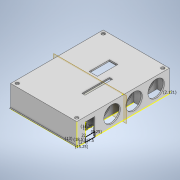
# Autodesk Inventor part: upper casing
Saved by Autodesk Inventor 2020 (Build 240168000, 168)
## iProperties
Created: 2019-06-23
Part Number: upper casing
Material: Generic
Document SubType Name: Modeling
Designer: jjsch
Density: 1 g/cm^3
Appearance: Default
Mass: 107.508 g
Surface Area: 832.789 cm^2
Volume: 107.508 cm^3
Author: jjsch
Autodesk Inventor part; units mm, degrees
ref_plane "YZ Plane" through (0, 0, 0) normal (1, 0, 0) x (0, 1, 0)
ref_plane "XZ Plane" through (0, 0, 0) normal (0, 1, 0) x (-1, 0, 0)
ref_plane "XY Plane" through (0, 0, 0) normal (0, 0, 1) x (1, 0, 0)
sketch "Sketch1" plane through (0, 0, 0) normal (0, 1, 0) x (-1, 0, 0)
  line L0 (-1.2, -80) -> (1.2, -80)
  line L1 (1.2, -80) -> (1.2, 80)
  line L2 (1.2, 80) -> (-1.2, 80)
  line L3 (-1.2, 80) -> (-1.2, -80)
  line L4 (-1.2, -80) -> (1.2, 80) construction
  line L5 (1.2, -80) -> (-1.2, 80) construction
  point P0 (0, 0)
  dimension "d0" = 2.4
  dimension "d1" = 160
  constraints: 12 end point, 2 midpoint, 2 parallel, 1 horizontal, 1 perpendicular
  measures "d0" distance of L2.end L1.end
  measures "d1" distance of L1.end L0.end
extrude "Extrusion1" add sketch "Sketch1" along normal blind 40
sketch "Sketch2" plane through (1.2, 0, 80) normal (1, 0, 0) x (0, 0, -1)
  line L0 (0, 0) -> (0, 40) projected
  line L1 (160, 0) -> (160, 40) projected
  circle A0 centre (60, 20) radius 15
  circle A1 centre (100, 20) radius 15
  circle A2 centre (140, 20) radius 15
  line L2 (28.75, 31.75) -> (11.25, 31.75)
  line L3 (11.25, 31.75) -> (11.25, 8.25)
  line L4 (11.25, 8.25) -> (28.75, 8.25)
  line L5 (28.75, 8.25) -> (28.75, 31.75)
  line L6 (28.75, 31.75) -> (11.25, 8.25) construction
  line L7 (11.25, 31.75) -> (28.75, 8.25) construction
  point P0 (80, 0)
  point P1 (20, 20)
  dimension "d4" = 60
  dimension "d5" = 20
  dimension "d6" = 40
  dimension "d7" = 20
  dimension "d8" = 30
  dimension "d9" = 30
  dimension "d10" = 30
  dimension "d11" = 17.5
  dimension "d12" = 23.5
  constraints: 12 end point, 3 centre point, 3 coincident, 2 midpoint, 2 parallel, 1 horizontal, 1 perpendicular
  measures "d4" distance from line of L0 point (60, 20)
  measures "d5" distance from line of L1 point (140, 20)
  measures "d6" distance of point (140, 20) point (100, 20)
  measures "d7" distance from line of L0 point (20, 20)
  measures "d8" diameter of A0
  measures "d9" diameter of A1
  measures "d10" diameter of A2
  measures "d11" distance of L4.end L3.end
  measures "d12" distance of L3.end L2.end
extrude "Extrusion2" cut sketch "Sketch2" against normal blind 40
sketch "Sketch3" plane through (1.2, 0, -80) normal (0, 0, -1) x (-1, 0, 0)
  line L0 (2.4, 0) -> (2.4, 40) projected
  point P0 (1.2, 0)
sketch "Sketch4" plane through (0, 40, 0) normal (0, 1, 0) x (1, 0, 0)
  line L0 (1.2, -80) -> (-118.8, -80)
  line L1 (-118.8, -80) -> (-118.8, 80)
  line L2 (-118.8, 80) -> (1.2, 80)
  line L3 (1.2, 80) -> (1.2, -80)
  point P0 (0, 0)
  dimension "d17" = 120
  dimension "d18" = 160
  constraints: 8 end point, 2 parallel, 1 horizontal, 1 perpendicular
  measures "d17" distance of L1.end L2.end
  measures "d18" distance of L0.end L1.end
extrude "Extrusion3" add sketch "Sketch4" against normal blind 2.4
sketch "Sketch5" plane through (-1.2, 0, -80) normal (-1, 0, 0) x (0, 0, 1)
  circle A0 centre (20, 20) radius 15 projected
  circle A1 centre (60, 20) radius 15 projected
  circle A2 centre (100, 20) radius 15 projected
  line L0 (160, 37.6) -> (0, 37.6) projected
  line L1 (9, 37.6) -> (31, 37.6)
  line L2 (31, 30.198) -> (31, 37.6)
  line L3 (9, 37.6) -> (9, 30.198)
  arc A3 (31, 30.198) -> (9, 30.198) centre (20, 20) ccw
  arc A4 (71, 30.198) -> (49, 30.198) centre (60, 20) ccw
  arc A5 (111, 30.198) -> (89, 30.198) centre (100, 20) ccw
  line L4 (49, 30.198) -> (49, 37.6)
  line L5 (49, 37.6) -> (71, 37.6)
  line L6 (71, 37.6) -> (71, 30.198)
  line L7 (89, 30.198) -> (89, 37.6)
  line L8 (89, 37.6) -> (111, 37.6)
  line L9 (111, 37.6) -> (111, 30.198)
  point P0 (80, 0)
  constraints: 18 end point, 12 point on circle, 6 point on line, 5 perpendicular, 3 centre point, 3 concentric, 1 parallel
extrude "Extrusion4" add sketch "Sketch5" along normal blind 28.6 contours A0 L3 L0 L2 | A1 L4 L0 L6 | A2 L7 L0 L9
sketch "Sketch6" plane through (-1.2, 0, -80) normal (-1, 0, 0) x (0, 0, 1)
  point P0 (80, 0)
sketch "Sketch7" plane through (-1.2, 0, -80) normal (-1, 0, 0) x (0, 0, 1)
  line L0 (160, 0) -> (160, 37.6) projected
  line L1 (129.75, 33.25) -> (129.75, 8.25)
  line L2 (129.75, 8.25) -> (150.25, 8.25)
  line L3 (150.25, 8.25) -> (150.25, 33.25)
  line L4 (151.5882, 33.25) -> (128.5882, 33.25)
  line L5 (131.25, 31.75) -> (148.75, 31.75) projected
  line L6 (150.25, 33.25) -> (129.75, 33.25)
  line L7 (151.25, 34.25) -> (151.25, 7.25)
  line L8 (151.25, 7.25) -> (128.75, 7.25)
  line L9 (128.75, 7.25) -> (128.75, 34.25)
  line L10 (128.75, 34.25) -> (151.25, 34.25)
  line L11 (148.75, 8.25) -> (131.25, 8.25) projected
  line L12 (131.25, 8.25) -> (131.25, 31.75) projected
  line L13 (148.75, 31.75) -> (148.75, 8.25) projected
  point P0 (80, 0)
  point P1 (129.75, 33.25)
  dimension "d25" = 20.5
  dimension "d26" = 25
  dimension "d27" = 23
  dimension "d129" = 1
  dimension "d158" = 1.5
  dimension "d159" = 1.5
  dimension "d160" = 1.5
  constraints: 18 end point, 2 parallel, 1 horizontal, 3 other
  measures "d25" distance of L2.end L1.end
  measures "d26" distance of L1.end L1.start
  measures "d27" distance of L4.end L4.start
  measures "d129" distance between parallel lines of L3 L7
  measures "d158" distance between parallel lines of L5 L6
  measures "d159" distance between parallel lines of L12 L1
  measures "d160" distance between parallel lines of L3 L13
extrude "Extrusion5" add sketch "Sketch7" along normal blind 1.5 contours L4 L9 L10 L7 | L1 L2 L3 L4 L7 L8 L9
sketch "Sketch12" plane through (1.2, 0, -80) normal (0, 0, -1) x (-1, 0, 0)
  line L0 (0, 40) -> (120, 40) projected
  line L1 (0, 40) -> (120, 40)
  line L2 (120, 40) -> (120, 0)
  line L3 (120, 0) -> (0, 0)
  line L4 (0, 0) -> (0, 40)
  point P0 (1.2, 0)
  dimension "d96" = 120
  constraints: 8 end point, 2 parallel, 1 horizontal, 1 perpendicular
  measures "d96" distance of L2.end L3.end
extrude "Extrusion10" add sketch "Sketch12" along normal blind 4
sketch "Sketch13" plane through (0, 37.6, 0) normal (0, -1, 0) x (1, 0, 0)
  point P0 (0, 0)
sketch "Sketch14" plane through (1.2, 0, 80) normal (0, 0, 1) x (1, 0, 0)
  line L0 (-120, 40) -> (-120, 37.6) projected
  line L1 (-2.4, 0) -> (0, 0) projected
  line L2 (-120, 40) -> (0, 40)
  line L3 (0, 40) -> (0, 0)
  line L4 (0, 0) -> (-120, 0)
  line L5 (-120, 0) -> (-120, 40)
  point P0 (-1.2, 0)
  constraints: 8 end point, 2 parallel, 1 horizontal, 1 perpendicular
extrude "Extrusion11" add sketch "Sketch14" along normal blind 4
sketch "Sketch15" plane through (1.2, 0, 68.75) normal (1, 0, 0) x (0, 0, -1)
  point P0 (68.75, 0)
sketch "Sketch16" plane through (0, 37.6, 0) normal (0, -1, 0) x (1, 0, 0)
  line L0 (-1.2, 80) -> (-118.8, 80) projected
  line L1 (-22.3, 80) -> (-17.3, 80)
  line L2 (-17.3, 80) -> (-17.3, -80)
  line L3 (-17.3, -80) -> (-22.3, -80)
  line L4 (-22.3, -80) -> (-22.3, 80)
  point P0 (0, 0)
  dimension "d47" = 5
  dimension "d48" = 160
  constraints: 8 end point, 2 parallel, 1 horizontal, 1 perpendicular, 1 point on line
  measures "d47" distance of L2.end L3.end
  measures "d48" distance of L1.end L2.end
extrude "Extrusion12" add sketch "Sketch16" along normal up to surface (37.6 mm away)
sketch "Sketch18" plane through (1.2, 0, 68.75) normal (1, 0, 0) x (0, 0, -1)
  point P0 (68.75, 0)
sketch "Sketch21" plane through (0, 37.6, 0) normal (0, -1, 0) x (1, 0, 0)
  line L0 (-1.2, -80) -> (-1.2, 80) projected
  line L1 (-17.3, -80) -> (-17.3, 80) projected
  line L2 (-1.2, -49) -> (-17.3, -49) projected
  line L3 (-1.2, -31) -> (-17.3, -31) projected
  line L4 (-17.3, -38) -> (-1.2, -38)
  line L5 (-1.2, -38) -> (-1.2, -42)
  line L6 (-1.2, -42) -> (-17.3, -42)
  line L7 (-17.3, -42) -> (-17.3, -38)
  line L8 (-17.3, -38) -> (-1.2, -42) construction
  line L9 (-1.2, -38) -> (-17.3, -42) construction
  point P0 (0, 0)
  point P1 (-9.25, -40)
  point P2 (-1.2, -2)
  point P3 (-17.3, -2)
  point P4 (-1.2, -38)
  dimension "d59" = 8.05
  dimension "d60" = 8.05
  dimension "d61" = 9
  dimension "d62" = 9
  dimension "d63" = 16.1
  dimension "d64" = 4
  constraints: 12 end point, 2 midpoint, 2 parallel, 1 horizontal, 1 perpendicular
  measures "d59" distance from line of L0 point (-9.25, -40)
  measures "d60" distance from line of L1 point (-9.25, -40)
  measures "d61" distance from line of L2 point (-9.25, -40)
  measures "d62" distance from line of L3 point (-9.25, -40)
  measures "d63" distance of L5.end L6.end
  measures "d64" distance of L4.end L5.end
extrude "Extrusion16" add sketch "Sketch21" along normal up to surface (37.6 mm away) contours L6 L1 L4 L0
sketch "Sketch22" plane through (0, 37.6, 0) normal (0, -1, 0) x (1, 0, 0)
  point P0 (0, 0)
sketch "Sketch23" plane through (0, 37.6, 0) normal (0, -1, 0) x (1, 0, 0)
  line L0 (-118.8, 80) -> (-118.8, -80) projected
  line L1 (-22.3, 80) -> (-118.8, 80) projected
  circle A0 centre (-66.3, 76.5) radius 3
  circle A1 centre (-115.3, 76.5) radius 3
  circle A2 centre (-115.3, 18.5) radius 3
  circle A3 centre (-66.3, 18.5) radius 3
  circle A4 centre (-66.3, 18.5) radius 1.375
  circle A5 centre (-115.3, 18.5) radius 1.375
  circle A6 centre (-115.3, 76.5) radius 1.375
  circle A7 centre (-66.3, 76.5) radius 1.375
  point P0 (0, 0)
  dimension "d67" = 58
  dimension "d68" = 58
  dimension "d69" = 49
  dimension "d70" = 3.5
  dimension "d71" = 3.5
  dimension "d72" = 6
  dimension "d73" = 6
  dimension "d74" = 6
  dimension "d75" = 6
  dimension "d78" = 2.75
  dimension "d79" = 2.75
  dimension "d80" = 2.75
  dimension "d81" = 2.75
  constraints: 8 centre point, 8 coincident, 2 vertical alignment, 1 horizontal alignment
  measures "d67" distance of point (-66.3, 18.5) point (-66.3, 76.5)
  measures "d68" distance of point (-115.3, 18.5) point (-115.3, 76.5)
  measures "d69" distance of point (-66.3, 18.5) point (-115.3, 18.5)
  measures "d70" distance from line of L0 point (-115.3, 76.5)
  measures "d71" distance from line of L1 point (-115.3, 76.5)
  measures "d72" diameter of A0
  measures "d73" diameter of A1
  measures "d74" diameter of A2
  measures "d75" diameter of A3
  measures "d78" diameter of A4
  measures "d79" diameter of A5
  measures "d80" diameter of A6
  measures "d81" diameter of A7
extrude "Extrusion17" add sketch "Sketch23" along normal blind 8
sketch "Sketch28" plane through (0, 0, 0) normal (0, -1, 0) x (1, 0, 0)
  point P0 (0, 0)
sketch "Sketch29" plane through (0, 37.6, 0) normal (0, -1, 0) x (1, 0, 0)
  circle A0 centre (-115.3, 18.5) radius 3 projected
  circle A1 centre (-66.3, 18.5) radius 3 projected
  circle A2 centre (-115.3, 76.5) radius 3 projected
  circle A3 centre (-66.3, 76.5) radius 3 projected
  line L0 (-1.2, -71) -> (-17.3, -71) projected
  line L1 (-29.8, -71) -> (-29.8, -49) projected
  line L2 (-29.8, -49) -> (-22.3, -49) projected
  line L3 (-1.2, -31) -> (-17.3, -31) projected
  line L4 (-29.8, -31) -> (-29.8, -9) projected
  line L5 (-29.8, -9) -> (-22.3, -9) projected
  line L6 (-1.2, 9) -> (-17.3, 9) projected
  line L7 (-29.8, 9) -> (-29.8, 31) projected
  line L8 (-29.8, 31) -> (-22.3, 31) projected
  line L9 (-1.2, 80) -> (-17.3, 80) projected
  line L10 (-118.8, 80) -> (-118.8, -80) projected
  line L11 (-118.8, -80) -> (-22.3, -80) projected
  line L12 (-35.8, -3) -> (-35.8, -37)
  line L13 (-35.8, -37) -> (-28.3, -37)
  line L14 (-28.3, -37) -> (-28.3, -43)
  line L15 (-28.3, -43) -> (-35.8, -43)
  line L16 (-35.8, -43) -> (-35.8, -74)
  line L17 (-35.8, -74) -> (-112.8, -74)
  line L18 (-112.8, -74) -> (-112.8, 74)
  line L19 (-112.8, 74) -> (-28.3, 74)
  line L20 (-28.3, 74) -> (-28.3, 37)
  line L21 (-28.3, 37) -> (-35.8, 37)
  line L22 (-35.8, 37) -> (-35.8, 3)
  line L23 (-35.8, 3) -> (-28.3, 3)
  line L24 (-28.3, 3) -> (-28.3, -3)
  line L25 (-28.3, -3) -> (-35.8, -3)
  line L26 (-112.8, -74) -> (-35.8, -74)
  line L27 (-35.8, -74) -> (-35.8, -6)
  line L28 (-35.8, -6) -> (-112.8, -6)
  line L29 (-112.8, -6) -> (-112.8, -74)
  line L30 (-66.3, -74) -> (-51.3, -74)
  line L31 (-51.3, -74) -> (-51.3, -6)
  line L32 (-51.3, -6) -> (-66.3, -6)
  line L33 (-66.3, -6) -> (-66.3, -74)
  line L34 (-51.3, -51.2056) -> (-36.3, -51.2056) construction
  line L35 (-118.8, -84) -> (1.2, -84) projected
  line L36 (-59.1553, -43) -> (-66.3, -43)
  line L37 (-59.1553, -43) -> (-51.3, -43)
  line L38 (-142.8, 0) -> (25.2, 0) projected
  line L39 (-17.3, 31) -> (-1.2, 31) projected
  line L40 (-1.2, -42) -> (-17.3, -42) projected
  line L41 (-17.3, -42) -> (-17.3, -49) projected
  line L42 (-17.3, -49) -> (-1.2, -49) projected
  line L43 (-1.2, -42) -> (-1.2, -49) projected
  line L44 (-17.3, -71) -> (-17.3, -80) projected
  line L45 (-17.3, -80) -> (-1.2, -80) projected
  line L46 (-1.2, -71) -> (-1.2, -80) projected
  line L47 (-17.3, 80) -> (-17.3, 31) projected
  line L48 (-17.3, -9) -> (-1.2, -9) projected
  line L49 (-1.2, 9) -> (-1.2, -9) projected
  line L50 (-1.2, 80) -> (-1.2, 31) projected
  line L51 (-17.3, 9) -> (-17.3, -9) projected
  line L52 (-17.3, -38) -> (-1.2, -38) projected
  line L53 (-1.2, -31) -> (-1.2, -38) projected
  line L54 (-17.3, -31) -> (-17.3, -38) projected
  line L55 (-22.3, 80) -> (-118.8, 80) projected
  line L56 (-22.3, -71) -> (-29.8, -71) projected
  line L57 (-22.3, -31) -> (-29.8, -31) projected
  line L58 (-22.3, 9) -> (-29.8, 9) projected
  line L59 (-22.3, 31) -> (-22.3, 80) projected
  line L60 (-22.3, -80) -> (-22.3, -71) projected
  line L61 (-22.3, -49) -> (-22.3, -31) projected
  line L62 (-22.3, -9) -> (-22.3, 9) projected
  point P0 (0, 0)
  point P1 (-66.3, -6)
  dimension "d97" = 6
  dimension "d98" = 15
  dimension "d110" = 41
  dimension "d118" = 6
  constraints: 50 end point, 6 point on line, 4 parallel, 3 horizontal, 3 perpendicular, 7 other
  measures "d97" distance between parallel lines of L4 L12
  measures "d98" distance of L32.end L31.end
  measures "d110" distance from line of L35 L36.start
  measures "d118" distance between parallel lines of L38 L28
extrude "Extrusion20" cut sketch "Sketch29" along normal mid plane 10 contours L28 L31 L37 L36 L33
sketch "Sketch30" plane through (0, 40, 0) normal (0, 1, 0) x (1, 0, 0)
  line L0 (-51.3, 43) -> (-51.3, 6) projected
  line L1 (-51.3, 6) -> (-66.3, 6) projected
  line L2 (-66.3, 6) -> (-66.3, 43) projected
  line L3 (1.2, 84) -> (1.2, -84) projected
  line L4 (-118.8, 84) -> (1.2, 84) projected
  line L5 (-118.8, 84) -> (-118.8, -84) projected
  line L6 (1.2, -84) -> (-118.8, -84) projected
  line L7 (-112.8, -78) -> (-112.8, 78)
  line L8 (-112.8, 78) -> (-4.8, 78)
  line L9 (-4.8, 78) -> (-4.8, -78)
  line L10 (-4.8, -78) -> (-112.8, -78)
  circle A0 centre (-112.8, -78) radius 3
  circle A1 centre (-112.8, 78) radius 3
  circle A2 centre (-4.8, -78) radius 3
  circle A3 centre (-4.8, 78) radius 3
  line L11 (-66.3, 43) -> (-51.3, 43) projected
  point P0 (0, 0)
  dimension "d101" = 6
  dimension "d102" = 6
  dimension "d103" = 6
  dimension "d104" = 6
  dimension "d105" = 6
  constraints: 8 coincident, 8 end point, 4 centre point, 3 other
  measures "d101" distance between parallel lines of L6 L10
  measures "d102" diameter of A0
  measures "d103" diameter of A1
  measures "d104" diameter of A2
  measures "d105" diameter of A3
sketch "Sketch31" plane through (0, 40, 0) normal (0, 1, 0) x (1, 0, 0)
  point P0 (0, 0)
extrude "Extrusion21" cut sketch "Sketch30" against normal blind 2 contours L10 A0 L7 | L7 A0 L10 | A1 L8 L7 | L7 L8 A1 | A2 L9 L10 | L10 L9 A2 | A3 L9 L8 | L8 L9 A3
sketch "Sketch32" plane through (0, 40, 0) normal (0, 1, 0) x (1, 0, 0)
  line L0 (1.2, 84) -> (1.2, -84) projected
  line L1 (-118.8, 84) -> (1.2, 84) projected
  line L2 (-32.842, -35) -> (-32.842, 15)
  line L3 (-32.842, 15) -> (-38.382, 15)
  line L4 (-38.382, 15) -> (-38.382, -35)
  line L5 (-38.382, -35) -> (-32.842, -35)
  point P0 (0, 0)
  dimension "d111" = 50
  dimension "d112" = 34.042
  dimension "d113" = 34.042
  dimension "d114" = 69
  dimension "d115" = 5.54
  constraints: 8 end point, 3 perpendicular
  measures "d111" distance of L2.end L2.start
  measures "d112" distance from line of L0 L2.start
  measures "d113" distance from line of L0 L2.end
  measures "d114" distance from line of L1 L2.end
  measures "d115" distance of L2.end L3.end
extrude "Extrusion22" cut sketch "Sketch32" against normal blind 10
sketch "Sketch33" plane through (0, 37.6, 0) normal (0, -1, 0) x (1, 0, 0)
  point P0 (0, 0)
sketch "Sketch34" plane through (0, 40, 0) normal (0, 1, 0) x (1, 0, 0)
  point P0 (0, 0)
sketch "Sketch42" plane through (-17.3, 37.6, 80) normal (1, 0, 0) x (0, 0, -1)
  line L0 (31, -26.35) -> (31, -3.6)
  line L1 (9, -3.6) -> (9, -26.35)
  line L2 (31, -3.6) -> (31, -4.35)
  line L3 (9, -3.6) -> (9, -4.35)
  line L4 (9, -4.35) -> (31, -4.35)
  line L5 (9, -26.35) -> (31, -26.35)
  line L6 (0, 0) -> (49, 0) projected
  line L7 (0, -37.6) -> (0, 0) projected
  line L8 (30.25, -4.35) -> (9.75, -4.35) projected
  line L9 (8.75, -3.35) -> (31.25, -3.35) projected
  point P0 (80, -37.6)
  point P1 (9, -4.35)
  dimension "d162" = 22
  dimension "d163" = 4.35
  dimension "d164" = 9
  dimension "d165" = 22
  dimension "d177" = 1
  constraints: 12 end point, 1 perpendicular, 1 point on line, 1 other
  measures "d162" distance between parallel lines of L5 L4
  measures "d163" distance between parallel lines of L4 L6
  measures "d164" distance between parallel lines of L1 L7
  measures "d165" distance between parallel lines of L0 L1
extrude "Extrusion30" cut sketch "Sketch42" against normal blind 10
sketch "Sketch43" plane through (-17.3, 37.6, 80) normal (1, 0, 0) x (0, 0, -1)
  line L0 (-0.75, -32.95) -> (2.65, -32.95)
  line L1 (2.65, -32.95) -> (2.65, -6.35)
  line L2 (2.65, -6.35) -> (-0.75, -6.35)
  line L3 (-0.75, -6.35) -> (-0.75, -32.95)
  line L4 (4.65, -34.95) -> (-2.75, -34.95)
  line L5 (-2.75, -34.95) -> (-2.75, -4.35)
  line L6 (-2.75, -4.35) -> (4.65, -4.35)
  line L7 (4.65, -4.35) -> (4.65, -34.95)
  line L8 (9, -4.35) -> (31, -4.35) projected
  point P0 (80, -37.6)
  point P1 (0.95, -27.95)
  point P2 (9, -26.35)
  point P3 (-4, -37.6)
  dimension "d168" = 8.05
  dimension "d169" = 1.6
  dimension "d170" = 3.4
  dimension "d172" = 2
  dimension "d173" = 3.25
  dimension "d174" = 1.25
  dimension "d178" = 0
  constraints: 16 end point, 4 parallel, 2 perpendicular, 1 horizontal, 3 other
  measures "d168" horizontal distance of point (0.95, -27.95) point (9, -26.35)
  measures "d169" vertical distance of point (9, -26.35) point (0.95, -27.95)
  measures "d170" distance of L2.end L1.end
  measures "d172" distance between parallel lines of L0 L4
  measures "d173" distance from line of point (-4, -37.6) L3
  measures "d174" distance from line of point (-4, -37.6) L5
  measures "d178" distance between parallel lines of L8 L6
extrude "Extrusion31" cut sketch "Sketch43" along normal mid plane 30 contours L3 L2 L1 L0 | L4 L5 L6 L7
sketch "Sketch44" plane through (-17.3, 37.6, 80) normal (1, 0, 0) x (0, 0, -1)
  circle A0 centre (60, -17.6) radius 15 projected
  circle A1 centre (100, -17.6) radius 15 projected
  circle A2 centre (140, -17.6) radius 15 projected
  point P0 (80, -37.6)
extrude "Extrusion32" cut sketch "Sketch44" against normal blind 30
sketch "Sketch45" plane through (1.2, 0, -84) normal (1, 0, 0) x (0, 0, -1)
  line L0 (-152.75, 31.75) -> (-152.75, 8.25) projected
  line L1 (-46, 0) -> (-164, 0) projected
  line L2 (-152.75, 8.25) -> (-135.25, 8.25)
  line L3 (-135.25, 8.25) -> (-135.25, 0)
  line L4 (-135.25, 0) -> (-152.75, 0)
  line L5 (-152.75, 0) -> (-152.75, 8.25)
  line L6 (-168, 0) -> (-168, 40) projected
  point P0 (-84, 0)
  dimension "d181" = 17.5
  dimension "d184" = 8.25
  dimension "d185" = 15.25
  constraints: 8 end point, 2 parallel, 1 horizontal, 1 perpendicular, 1 point on line
  measures "d181" distance of L3.end L4.end
  measures "d184" distance of L2.end L3.end
  measures "d185" distance from line of L4.end L6
extrude "Extrusion33" cut sketch "Sketch45" against normal blind 30
sketch "Sketch46" plane through (0, 0, 0) normal (0, -1, 0) x (1, 0, 0)
  line L0 (-1.2, 68.75) -> (-1.2, 80) projected
  line L1 (1.2, 84) -> (1.2, 68.75) projected
  point P0 (0, 0)
  dimension "d186" = 2.4
  measures "d186" distance between parallel lines of L0 L1
sketch "Sketch47" plane through (0, 0, 0) normal (0, -1, 0) x (1, 0, 0)
  line L0 (-0.6375, 52.5) -> (0.6375, 52.5)
  line L1 (0.6375, 52.5) -> (0.6375, 50)
  line L2 (0.6375, 50) -> (-0.6375, 50)
  line L3 (-0.6375, 50) -> (-0.6375, 52.5)
  line L4 (1.2, 51.25) -> (-1.2, 51.25) projected
  line L5 (-0.6375, 52.5) -> (0.6375, 50) construction
  line L6 (0.6375, 52.5) -> (-0.6375, 50) construction
  line L7 (-0.6375, 70) -> (0.6375, 70)
  line L8 (0.6375, 70) -> (0.6375, 67.5)
  line L9 (0.6375, 67.5) -> (-0.6375, 67.5)
  line L10 (-0.6375, 67.5) -> (-0.6375, 70)
  line L11 (-1.2, 68.75) -> (1.2, 68.75) projected
  line L12 (-0.6375, 70) -> (0.6375, 67.5) construction
  line L13 (0.6375, 70) -> (-0.6375, 67.5) construction
  point P0 (0, 0)
  point P1 (0, 51.25)
  point P2 (0, 68.75)
  point P3 (0.6375, 51.25)
  point P4 (-0.6375, 51.25)
  point P5 (-0.6375, 68.75)
  point P6 (0.6375, 68.75)
  dimension "d187" = 1.275
  dimension "d188" = 2.5
  dimension "d189" = 1.275
  dimension "d190" = 2.5
  constraints: 24 end point, 6 midpoint, 4 parallel, 2 horizontal, 2 perpendicular
  measures "d187" distance of L1.end L2.end
  measures "d188" distance of L0.end L1.end
  measures "d189" distance of L8.end L9.end
  measures "d190" distance of L7.end L8.end
extrude "Extrusion34" cut sketch "Sketch47" against normal blind 8.25 contours L4 L1 L2 L3 | L7 L8 L11 L10
sketch "Sketch48" plane through (-17.3, 37.6, 80) normal (1, 0, 0) x (0, 0, -1)
  line L0 (31, -4.35) -> (31, -26.35) projected
  line L1 (9, -26.35) -> (9, -4.35) projected
  line L2 (9, -4.35) -> (9, -26.35) projected
  line L3 (118, -37.6) -> (28.75, -37.6) projected
  line L4 (9, -26.35) -> (31, -26.35)
  line L5 (31, -26.35) -> (31, -37.6)
  line L6 (31, -37.6) -> (9, -37.6)
  line L7 (9, -37.6) -> (9, -26.35)
  point P0 (80, -37.6)
  point P1 (28.75, -37.6)
  dimension "d193" = 11.25
  dimension "d194" = 22
  constraints: 8 end point, 2 parallel, 1 horizontal, 1 perpendicular, 1 point on line
  measures "d193" distance of L4.end L5.end
  measures "d194" distance of L5.end L6.end
extrude "Extrusion35" cut sketch "Sketch48" against normal blind 5
sketch "Sketch49" plane through (0, 0, 0) normal (0, -1, 0) x (1, 0, 0)
  line L0 (-22.3, 49) -> (-22.3, -80) projected
  line L1 (-17.3, -38) -> (-17.3, 49) projected
  line L2 (-118.8, 84) -> (1.2, 84) projected
  line L3 (-22.3, 71) -> (-17.3, 71) projected
  line L4 (1.2, 84) -> (1.2, 68.75) projected
  line L5 (-17.3, 71) -> (-17.3, 80) projected
  point P0 (0, 0)
  dimension "d197" = 5
  dimension "d198" = 13
  dimension "d199" = 18.5
  measures "d197" distance between parallel lines of L0 L1
  measures "d198" distance between parallel lines of L2 L3
  measures "d199" distance between parallel lines of L4 L5
sketch "Sketch50" plane through (0, 0, 0) normal (0, -1, 0) x (1, 0, 0)
  line L0 (-17.3, 49) -> (-22.3, 49) projected
  line L1 (-22.3, 71) -> (-17.3, 71) projected
  line L2 (-18.475, 45) -> (-21.125, 45)
  line L3 (-21.125, 45) -> (-21.125, 53)
  line L4 (-21.125, 53) -> (-18.475, 53)
  line L5 (-18.475, 53) -> (-18.475, 45)
  line L6 (-18.475, 45) -> (-21.125, 53) construction
  line L7 (-21.125, 45) -> (-18.475, 53) construction
  line L8 (-18.475, 75) -> (-21.125, 75)
  line L9 (-21.125, 75) -> (-21.125, 67)
  line L10 (-21.125, 67) -> (-18.475, 67)
  line L11 (-18.475, 67) -> (-18.475, 75)
  line L12 (-18.475, 75) -> (-21.125, 67) construction
  line L13 (-21.125, 75) -> (-18.475, 67) construction
  point P0 (0, 0)
  point P1 (-19.8, 49)
  point P2 (-19.8, 71)
  dimension "d200" = 2.65
  dimension "d201" = 8
  dimension "d202" = 2.65
  dimension "d203" = 8
  constraints: 24 end point, 6 midpoint, 4 parallel, 2 horizontal, 2 perpendicular
  measures "d200" distance of L3.end L4.end
  measures "d201" distance of L2.end L3.end
  measures "d202" distance of L10.end L9.end
  measures "d203" distance of L9.end L8.end
extrude "Extrusion36" cut sketch "Sketch50" against normal blind 11.25
sketch "Sketch51" plane through (1.2, 0, 68.75) normal (1, 0, 0) x (0, 0, -1)
  line L0 (17.5, 0) -> (152.75, 0) projected
  line L1 (152.75, 0) -> (154.8713, 2.1213)
  line L2 (152.75, 0) -> (155.75, 0) construction
  line L3 (154.8713, 2.1213) -> (152.75, 2.1213)
  line L4 (152.75, 40) -> (152.75, 0) projected
  line L5 (152.75, 2.1213) -> (152.75, 0)
  point P0 (68.75, 0)
  dimension "d206" = 3
  dimension "d207" = 45
  constraints: 8 end point, 1 collinear, 1 equal length, 1 horizontal
  measures "d206" distance of L0.end L1.end
  measures "d207" angle of L2 L1
extrude "Extrusion37" add sketch "Sketch51" against normal up to surface (120 mm away)
ref_plane "Work Plane3" through (1.2, 0, 0) normal (0, 0, 1) x (1, 0, 0)
mirror "Mirror3" about plane through (1.2, 0, 0) normal (0, 0, 1) of "Extrusion37"
sketch "Sketch52" plane through (1.2, 0, 68.75) normal (1, 0, 0) x (0, 0, -1)
  line L0 (17.5, 0) -> (152.75, 0) projected
  line L1 (154.8713, 2.1213) -> (152.75, 2.1213) projected
  point P0 (68.75, 0)
  dimension "d210" = 2.121
sketch "Sketch53" plane through (0, 0, 0) normal (0, -1, 0) x (1, 0, 0)
  line L0 (-1.2, -80) -> (-1.2, -42) projected
  line L1 (-1.2, -80) -> (-17.3, -80) projected
  line L2 (-17.3, -80) -> (-17.3, -42) projected
  line L3 (-17.3, -42) -> (-1.2, -42) projected
  line L4 (-18.475, 49) -> (-18.475, 45) projected
  line L5 (-18.475, 45) -> (-21.125, 45) projected
  line L6 (-21.125, 45) -> (-21.125, 49) projected
  line L7 (-21.125, 49) -> (-22.3, 49) projected
  line L8 (-22.3, 49) -> (-22.3, -80) projected
  line L9 (-22.3, -80) -> (-118.8, -80) projected
  line L10 (-118.8, -80) -> (-118.8, -84) projected
  line L11 (1.2, -84) -> (-118.8, -84) projected
  line L12 (1.2, 51.25) -> (1.2, -84) projected
  line L13 (1.2, 51.25) -> (0.6375, 51.25) projected
  line L14 (0.6375, 51.25) -> (0.6375, 50) projected
  line L15 (0.6375, 50) -> (-0.6375, 50) projected
  line L16 (-0.6375, 50) -> (-0.6375, 51.25) projected
  line L17 (-0.6375, 51.25) -> (-1.2, 51.25) projected
  line L18 (-1.2, -38) -> (-1.2, 51.25) projected
  line L19 (-1.2, -38) -> (-17.3, -38) projected
  line L20 (-17.3, -38) -> (-17.3, 49) projected
  line L21 (-17.3, 49) -> (-18.475, 49) projected
  line L22 (-18.8, 43.5) -> (-18.8, -39.5)
  line L23 (-18.8, -39.5) -> (-0.3, -39.5)
  line L24 (-0.3, -39.5) -> (-0.3, -82.5)
  line L25 (-0.3, -82.5) -> (-117.3, -82.5)
  line L26 (-117.3, -82.5) -> (-117.3, -81.5)
  line L27 (-117.3, -81.5) -> (-20.8, -81.5)
  line L28 (-20.8, -81.5) -> (-20.8, 43.5)
  line L29 (-20.8, 43.5) -> (-18.8, 43.5)
  line L30 (-18.8, 43.5) -> (-20.8, 43.5)
  line L31 (-20.8, 43.5) -> (-20.8, -82.5)
  line L32 (-20.8, -82.5) -> (-18.8, -82.5)
  line L33 (-18.8, -82.5) -> (-18.8, 43.5)
  point P0 (0, 0)
  point P1 (-18.8, -39.5)
  dimension "d211" = 1.5
  constraints: 24 end point, 2 parallel, 1 horizontal, 1 perpendicular, 1 point on line, 7 other
  measures "d211" distance between parallel lines of L20 L22
extrude "Extrusion38" cut sketch "Sketch53" against normal up to surface (37.6 mm away) contours L22 L33 L25 L31 L28 L29
body "Solid1"
